Autodesk Fusion 360 part; units mm, degrees
(part 4 of 7)
  arc A299 (52.4822, -27.8177) -> (51.9822, -28.3177) centre (52.4822, -28.3177) ccw
  arc A300 (179.3389, -62.3677) -> (179.8389, -62.8677) centre (179.8389, -62.3677) ccw
  arc A301 (113.1072, -3.7177) -> (113.6072, -3.2177) centre (113.1072, -3.2177) ccw
  arc A302 (-38.5053, -60.3677) -> (-38.0053, -60.8677) centre (-38.0053, -60.3677) ccw
  arc A303 (157.2572, -84.9677) -> (156.7572, -85.4677) centre (157.2572, -85.4677) ccw
  arc A304 (94.5572, 9.7823) -> (94.0572, 10.2823) centre (94.0572, 9.7823) ccw
  arc A305 (46.9322, -28.3177) -> (46.4322, -27.8177) centre (46.4322, -28.3177) ccw
  arc A306 (-52.2928, 10.2823) -> (-52.7928, 9.7823) centre (-52.2928, 9.7823) ccw
  arc A307 (-70.2491, -60.8677) -> (-69.7491, -60.3677) centre (-70.2491, -60.3677) ccw
  arc A308 (-14.1928, -8.7677) -> (-14.6928, -9.2677) centre (-14.1928, -9.2677) ccw
  arc A309 (189.8072, -85.4677) -> (189.3072, -84.9677) centre (189.3072, -85.4677) ccw
  arc A310 (-34.5303, -79.9177) -> (-34.0303, -79.4177) centre (-34.5303, -79.4177) ccw
  arc A311 (75.5072, -9.2677) -> (75.0072, -8.7677) centre (75.0072, -9.2677) ccw
  line L329 (113.6072, 9.7823) -> (113.6072, -3.2177)
  arc A312 (-0.6928, 9.7823) -> (-1.1928, 10.2823) centre (-1.1928, 9.7823) ccw
  arc A313 (208.8572, -85.4677) -> (208.3572, -84.9677) centre (208.3572, -85.4677) ccw
  arc A314 (136.9197, -79.9177) -> (137.4197, -79.4177) centre (136.9197, -79.4177) ccw
  arc A315 (65.9822, -28.3177) -> (65.4822, -27.8177) centre (65.4822, -28.3177) ccw
  arc A316 (75.0072, -3.7177) -> (75.5072, -3.2177) centre (75.0072, -3.2177) ccw
  arc A317 (-15.9491, -100.4677) -> (-15.4491, -100.9677) centre (-15.4491, -100.4677) ccw
  line L330 (114.3947, -60.8677) -> (127.3947, -60.8677)
  arc A318 (195.3572, -84.9677) -> (194.8572, -85.4677) centre (195.3572, -85.4677) ccw
  arc A319 (123.4197, -79.4177) -> (123.9197, -79.9177) centre (123.9197, -79.4177) ccw
  arc A320 (-9.4303, -65.9177) -> (-9.9303, -66.4177) centre (-9.4303, -66.4177) ccw
  line L331 (94.5572, -9.2677) -> (94.5572, -22.2677)
  line L332 (4.3572, -9.2677) -> (4.3572, -22.2677)
  line L333 (-74.5116, -85.4677) -> (-74.5116, -98.4677)
  arc A321 (30.5509, -98.4677) -> (31.0509, -98.9677) centre (31.0509, -98.4677) ccw
  arc A322 (42.4572, -22.2677) -> (42.9572, -22.7677) centre (42.9572, -22.2677) ccw
  arc A323 (-15.4491, -85.9677) -> (-15.9491, -86.4677) centre (-15.4491, -86.4677) ccw
  line L334 (-61.8178, -41.8177) -> (-48.8178, -41.8177)
  line L335 (158.3442, -9.7677) -> (164.3442, -9.7677)
  line L336 (-63.5486, -67.4177) -> (-63.5486, -81.4177)
  line L337 (194.8572, -85.4677) -> (194.8572, -98.4677)
  line L338 (42.1697, -66.4177) -> (42.1697, -79.4177)
  line L339 (99.6072, 9.7823) -> (99.6072, -3.2177)
  arc A324 (100.1072, -8.7677) -> (99.6072, -9.2677) centre (100.1072, -9.2677) ccw
  arc A325 (-57.8428, -9.2677) -> (-58.3428, -8.7677) centre (-58.3428, -9.2677) ccw
  arc A326 (-34.0303, -66.4177) -> (-34.5303, -65.9177) centre (-34.5303, -66.4177) ccw
  arc A327 (-88.5116, -98.4677) -> (-88.0116, -98.9677) centre (-88.0116, -98.4677) ccw
  arc A328 (123.9197, -65.9177) -> (123.4197, -66.4177) centre (123.9197, -66.4177) ccw
  line L340 (75.5072, -9.2677) -> (75.5072, -22.2677)
  line L341 (38.1947, -46.8677) -> (51.1947, -46.8677)
  arc A329 (176.3072, -65.9177) -> (175.8072, -66.4177) centre (176.3072, -66.4177) ccw
  line L342 (-88.0116, -84.9677) -> (-75.0116, -84.9677)
  line L343 (-40.8866, -85.4677) -> (-40.8866, -98.4677)
  line L344 (118.3697, -66.4177) -> (118.3697, -79.4177)
  arc A330 (151.2072, -3.7177) -> (151.7072, -3.2177) centre (151.2072, -3.2177) ccw
  arc A331 (22.6197, -79.9177) -> (23.1197, -79.4177) centre (22.6197, -79.4177) ccw
  arc A332 (-80.4246, -67.4177) -> (-80.9246, -66.9177) centre (-80.9246, -67.4177) ccw
  line L345 (18.3572, -9.2677) -> (18.3572, -22.2677)
  line L346 (-26.8866, -85.4677) -> (-26.8866, -98.4677)
  arc A333 (155.4629, -62.3677) -> (155.9629, -62.8677) centre (155.9629, -62.3677) ccw
  arc A334 (119.1572, -8.7677) -> (118.6572, -9.2677) centre (119.1572, -9.2677) ccw
  arc A335 (-39.2928, -3.7177) -> (-38.7928, -3.2177) centre (-39.2928, -3.2177) ccw
  line L347 (31.0509, -98.9677) -> (44.0509, -98.9677)
  line L348 (-64.9866, -66.4177) -> (-64.9866, -79.4177)
  line L349 (-87.4246, -67.4177) -> (-87.4246, -81.4177)
  arc A336 (17.8572, -22.7677) -> (18.3572, -22.2677) centre (17.8572, -22.2677) ccw
  arc A337 (-83.7491, -60.3677) -> (-83.2491, -60.8677) centre (-83.2491, -60.3677) ccw
  arc A338 (108.3447, -60.8677) -> (108.8447, -60.3677) centre (108.3447, -60.3677) ccw
  line L350 (176.3072, -65.9177) -> (189.3072, -65.9177)
  line L351 (151.7072, 9.7823) -> (151.7072, -3.2177)
  line L352 (-15.9491, -86.4677) -> (-15.9491, -100.4677)
  arc A339 (-52.2928, -8.7677) -> (-52.7928, -9.2677) centre (-52.2928, -9.2677) ccw
  line L353 (-15.4491, -100.9677) -> (-9.4491, -100.9677)
  line L354 (44.5509, -85.4677) -> (44.5509, -98.4677)
  arc A340 (57.2447, -46.8677) -> (56.7447, -47.3677) centre (57.2447, -47.3677) ccw
  arc A341 (85.3197, -79.4177) -> (85.8197, -79.9177) centre (85.8197, -79.4177) ccw
  line L355 (-48.0303, -66.4177) -> (-48.0303, -79.4177)
  line L356 (80.5572, -9.2677) -> (80.5572, -22.2677)
  arc A342 (-15.4803, -79.9177) -> (-14.9803, -79.4177) centre (-15.4803, -79.4177) ccw
  line L357 (56.4572, -9.2677) -> (56.4572, -22.2677)
  line L358 (138.2072, 10.2823) -> (151.2072, 10.2823)
  arc A343 (-74.5116, -85.4677) -> (-75.0116, -84.9677) centre (-75.0116, -85.4677) ccw
  line L359 (156.7572, 9.7823) -> (156.7572, -3.2177)
  line L360 (47.2197, -66.4177) -> (47.2197, -79.4177)
  arc A344 (9.1197, -79.4177) -> (9.6197, -79.9177) centre (9.6197, -79.4177) ccw
  arc A345 (44.0509, -98.9677) -> (44.5509, -98.4677) centre (44.0509, -98.4677) ccw
  line L361 (-50.6991, -85.4677) -> (-50.6991, -98.4677)
  arc A346 (118.6572, -3.2177) -> (119.1572, -3.7177) centre (119.1572, -3.2177) ccw
  line L362 (100.1072, -8.7677) -> (113.1072, -8.7677)
  line L363 (104.3697, -66.4177) -> (104.3697, -79.4177)
  arc A347 (4.8572, -8.7677) -> (4.3572, -9.2677) centre (4.8572, -9.2677) ccw
  line L364 (186.3389, -48.3677) -> (186.3389, -62.3677)
  arc A348 (99.6072, -3.2177) -> (100.1072, -3.7177) centre (100.1072, -3.2177) ccw
  arc A349 (118.3697, -66.4177) -> (117.8697, -65.9177) centre (117.8697, -66.4177) ccw
  line L365 (28.6697, -65.9177) -> (41.6697, -65.9177)
  arc A350 (60.7197, -79.9177) -> (61.2197, -79.4177) centre (60.7197, -79.4177) ccw
  arc A351 (151.7072, 9.7823) -> (151.2072, 10.2823) centre (151.2072, 9.7823) ccw
  arc A352 (51.1947, -60.8677) -> (51.6947, -60.3677) centre (51.1947, -60.3677) ccw
  arc A353 (117.8697, -79.9177) -> (118.3697, -79.4177) centre (117.8697, -79.4177) ccw
  arc A354 (-40.8866, -98.4677) -> (-40.3866, -98.9677) centre (-40.3866, -98.4677) ccw
  arc A355 (-33.2428, 10.2823) -> (-33.7428, 9.7823) centre (-33.2428, 9.7823) ccw
  arc A356 (66.2697, -79.4177) -> (66.7697, -79.9177) centre (66.7697, -79.4177) ccw
  line L366 (157.2572, 10.2823) -> (170.2572, 10.2823)
  arc A357 (176.3072, -84.9677) -> (175.8072, -85.4677) centre (176.3072, -85.4677) ccw
  arc A358 (-64.1991, -84.9677) -> (-64.6991, -85.4677) centre (-64.1991, -85.4677) ccw
  arc A359 (-64.9866, -66.4177) -> (-65.4866, -65.9177) centre (-65.4866, -66.4177) ccw
  line L367 (-80.4246, -67.4177) -> (-80.4246, -81.4177)
  arc A360 (3.5697, -79.9177) -> (4.0697, -79.4177) centre (3.5697, -79.4177) ccw
  arc A361 (-58.3428, -3.7177) -> (-57.8428, -3.2177) centre (-58.3428, -3.2177) ccw
  arc A362 (-28.4803, -65.9177) -> (-28.9803, -66.4177) centre (-28.4803, -66.4177) ccw
  line L368 (100.1072, -3.7177) -> (113.1072, -3.7177)
  arc A363 (-5.9553, -60.8677) -> (-5.4553, -60.3677) centre (-5.9553, -60.3677) ccw
  arc A364 (-88.0116, -84.9677) -> (-88.5116, -85.4677) centre (-88.0116, -85.4677) ccw
  line L369 (37.4072, -9.2677) -> (37.4072, -22.2677)
  arc A365 (51.6947, -47.3677) -> (51.1947, -46.8677) centre (51.1947, -47.3677) ccw
  arc A366 (19.1447, -46.8677) -> (18.6447, -47.3677) centre (19.1447, -47.3677) ccw
  arc A367 (51.9822, -41.3177) -> (52.4822, -41.8177) centre (52.4822, -41.3177) ccw
  line L370 (99.3197, -66.4177) -> (99.3197, -79.4177)
  line L371 (-19.7428, -9.2677) -> (-19.7428, -22.2677)
  line L372 (47.7197, -65.9177) -> (60.7197, -65.9177)
  line L373 (52.4822, -41.8177) -> (65.4822, -41.8177)
  line L374 (52.4822, -27.8177) -> (65.4822, -27.8177)
  arc A368 (170.2572, -3.7177) -> (170.7572, -3.2177) centre (170.2572, -3.2177) ccw
  line L375 (189.8072, 9.7823) -> (189.8072, -3.2177)
  arc A369 (180.2822, -9.2677) -> (179.7822, -8.7677) centre (179.7822, -9.2677) ccw
  line L376 (208.8572, 9.7823) -> (208.8572, -3.2177)
  arc A370 (208.8572, 9.7823) -> (208.3572, 10.2823) centre (208.3572, 9.7823) ccw
  arc A371 (195.3572, 10.2823) -> (194.8572, 9.7823) centre (195.3572, 9.7823) ccw
  arc A372 (182.2202, -9.7677) -> (181.7202, -10.2677) centre (182.2202, -10.2677) ccw
  arc A373 (208.3572, -3.7177) -> (208.8572, -3.2177) centre (208.3572, -3.2177) ccw
  line L377 (195.3572, 10.2823) -> (208.3572, 10.2823)
  line L378 (195.3572, -3.7177) -> (208.3572, -3.7177)
  line L379 (176.3072, -3.7177) -> (189.3072, -3.7177)
  line L380 (176.3072, 10.2823) -> (189.3072, 10.2823)
  arc A374 (175.8072, -3.2177) -> (176.3072, -3.7177) centre (176.3072, -3.2177) ccw
  arc A375 (195.3572, -8.7677) -> (194.8572, -9.2677) centre (195.3572, -9.2677) ccw
  arc A376 (176.3072, 10.2823) -> (175.8072, 9.7823) centre (176.3072, 9.7823) ccw
  line L381 (195.3572, -8.7677) -> (208.3572, -8.7677)
  arc A377 (170.7572, 9.7823) -> (170.2572, 10.2823) centre (170.2572, 9.7823) ccw
  arc A378 (177.9009, -47.3677) -> (177.4009, -46.8677) centre (177.4009, -47.3677) ccw
  arc A379 (208.8572, -28.3177) -> (208.3572, -27.8177) centre (208.3572, -28.3177) ccw
  arc A380 (171.5447, -27.8177) -> (171.0447, -28.3177) centre (171.5447, -28.3177) ccw
  line L382 (146.9447, -47.3677) -> (146.9447, -60.3677)
  arc A381 (188.2202, -24.7677) -> (188.7202, -24.2677) centre (188.2202, -24.2677) ccw
  line L383 (171.0447, -28.3177) -> (171.0447, -41.3177)
  line L384 (-5.4553, -47.3677) -> (-5.4553, -60.3677)
  arc A382 (195.3572, -27.8177) -> (194.8572, -28.3177) centre (195.3572, -28.3177) ccw
  arc A383 (162.4629, -48.3677) -> (161.9629, -47.8677) centre (161.9629, -48.3677) ccw
  line L385 (208.8572, -9.2677) -> (208.8572, -22.2677)
  line L386 (132.9447, -47.3677) -> (132.9447, -60.3677)
  arc A384 (195.3572, -46.8677) -> (194.8572, -47.3677) centre (195.3572, -47.3677) ccw
  line L387 (180.2822, -9.2677) -> (180.2822, -22.2677)
  arc A385 (186.3389, -48.3677) -> (185.8389, -47.8677) centre (185.8389, -48.3677) ccw
  line L388 (181.7202, -10.2677) -> (181.7202, -24.2677)
  line L389 (-24.5053, -47.3677) -> (-24.5053, -60.3677)
  line L390 (-113.7226, -118.8427) -> (-113.7226, 57.4273)
  line L391 (42.9572, 10.2823) -> (55.9572, 10.2823)
  line L392 (188.7202, -10.2677) -> (188.7202, -24.2677)
  arc A386 (37.4072, -9.2677) -> (36.9072, -8.7677) centre (36.9072, -9.2677) ccw
  line L393 (-43.5553, -47.3677) -> (-43.5553, -60.3677)
  line L394 (194.8572, -9.2677) -> (194.8572, -22.2677)
  line L395 (75.7947, -47.3677) -> (75.7947, -60.3677)
  line L396 (-57.5553, -47.3677) -> (-57.5553, -60.3677)
  line L397 (194.8572, -47.3677) -> (194.8572, -60.3677)
  line L398 (42.9572, -3.7177) -> (55.9572, -3.7177)
  line L399 (177.9009, -47.3677) -> (177.9009, -60.3677)
  arc A387 (55.9572, -3.7177) -> (56.4572, -3.2177) centre (55.9572, -3.2177) ccw
  arc A388 (56.4572, 9.7823) -> (55.9572, 10.2823) centre (55.9572, 9.7823) ccw
  arc A389 (17.8572, -3.7177) -> (18.3572, -3.2177) centre (17.8572, -3.2177) ccw
  line L400 (194.8572, 9.7823) -> (194.8572, -3.2177)
  arc A390 (194.8572, -3.2177) -> (195.3572, -3.7177) centre (195.3572, -3.2177) ccw
  line L401 (175.8072, 9.7823) -> (175.8072, -3.2177)
  arc A391 (188.7202, -10.2677) -> (188.2202, -9.7677) centre (188.2202, -10.2677) ccw
  arc A392 (208.8572, -47.3677) -> (208.3572, -46.8677) centre (208.3572, -47.3677) ccw
  line L402 (171.5447, -27.8177) -> (184.5447, -27.8177)
  arc A393 (179.7822, -22.7677) -> (180.2822, -22.2677) centre (179.7822, -22.2677) ccw
  line L403 (163.9009, -47.3677) -> (163.9009, -60.3677)
  line L404 (195.3572, -46.8677) -> (208.3572, -46.8677)
  line L405 (94.8447, -47.3677) -> (94.8447, -60.3677)
  line L406 (182.2202, -24.7677) -> (188.2202, -24.7677)
  line L407 (179.8389, -47.8677) -> (185.8389, -47.8677)
  line L408 (208.8572, -28.3177) -> (208.8572, -41.3177)
  arc A394 (184.5447, -41.8177) -> (185.0447, -41.3177) centre (184.5447, -41.3177) ccw
  arc A395 (185.0447, -28.3177) -> (184.5447, -27.8177) centre (184.5447, -28.3177) ccw
  arc A396 (189.3072, -3.7177) -> (189.8072, -3.2177) centre (189.3072, -3.2177) ccw
  arc A397 (189.8072, 9.7823) -> (189.3072, 10.2823) centre (189.3072, 9.7823) ccw
  line L409 (182.2202, -9.7677) -> (188.2202, -9.7677)
  line L410 (47.7197, -79.9177) -> (60.7197, -79.9177)
  line L411 (57.2447, -46.8677) -> (70.2447, -46.8677)
  line L412 (-113.7226, 57.4273) -> (228.9474, 57.4273)
  line L413 (18.6447, -47.3677) -> (18.6447, -60.3677)
  line L414 (89.7947, -47.3677) -> (89.7947, -60.3677)
  arc A398 (36.9072, -3.7177) -> (37.4072, -3.2177) centre (36.9072, -3.2177) ccw
  arc A399 (42.9572, -8.7677) -> (42.4572, -9.2677) centre (42.9572, -9.2677) ccw
  line L415 (56.7447, -47.3677) -> (56.7447, -60.3677)
  line L416 (51.6947, -47.3677) -> (51.6947, -60.3677)
  line L417 (-0.4053, -47.3677) -> (-0.4053, -60.3677)
  line L418 (208.8572, -47.3677) -> (208.8572, -60.3677)
  arc A400 (37.4072, 9.7823) -> (36.9072, 10.2823) centre (36.9072, 9.7823) ccw
  line L419 (13.5947, -47.3677) -> (13.5947, -60.3677)
  line L420 (-83.7491, -47.3677) -> (-83.7491, -60.3677)
  line L421 (-38.5053, -47.3677) -> (-38.5053, -60.3677)
  line L422 (127.8947, -47.3677) -> (127.8947, -60.3677)
  line L423 (37.6947, -47.3677) -> (37.6947, -60.3677)
  arc A401 (23.9072, -8.7677) -> (23.4072, -9.2677) centre (23.9072, -9.2677) ccw
  arc A402 (179.8389, -47.8677) -> (179.3389, -48.3677) centre (179.8389, -48.3677) ccw
  line L424 (70.7447, -47.3677) -> (70.7447, -60.3677)
  line L425 (-19.4553, -47.3677) -> (-19.4553, -60.3677)
  arc A403 (56.4572, -9.2677) -> (55.9572, -8.7677) centre (55.9572, -9.2677) ccw
  line L426 (113.8947, -47.3677) -> (113.8947, -60.3677)
  arc A404 (23.9072, 10.2823) -> (23.4072, 9.7823) centre (23.9072, 9.7823) ccw
  line L427 (108.8447, -47.3677) -> (108.8447, -60.3677)
  line L428 (-69.7491, -47.3677) -> (-69.7491, -60.3677)
  line L429 (32.6447, -47.3677) -> (32.6447, -60.3677)
  line L430 (-18.9553, -60.8677) -> (-5.9553, -60.8677)
  line L431 (-23.7178, -27.8177) -> (-10.7178, -27.8177)
  line L432 (228.9474, 57.4273) -> (228.9474, -118.8427)
  arc A405 (18.3572, -9.2677) -> (17.8572, -8.7677) centre (17.8572, -9.2677) ccw
  line L433 (-28.4803, -65.9177) -> (-15.4803, -65.9177)
  line L434 (-33.2428, 10.2823) -> (-20.2428, 10.2823)
  arc A406 (42.4572, -3.2177) -> (42.9572, -3.7177) centre (42.9572, -3.2177) ccw
  line L435 (23.9072, -8.7677) -> (36.9072, -8.7677)
  line L436 (-33.2428, -8.7677) -> (-20.2428, -8.7677)
  line L437 (42.4572, 9.7823) -> (42.4572, -3.2177)
  line L438 (-23.7178, -41.8177) -> (-10.7178, -41.8177)
  line L439 (18.3572, 9.7823) -> (18.3572, -3.2177)
  line L440 (119.1572, -8.7677) -> (132.1572, -8.7677)
  arc A407 (155.9629, -47.8677) -> (155.4629, -48.3677) centre (155.9629, -48.3677) ccw
  line L441 (-28.4803, -79.9177) -> (-15.4803, -79.9177)
  line L442 (123.9197, -79.9177) -> (136.9197, -79.9177)
  line L443 (-57.0553, -60.8677) -> (-44.0553, -60.8677)
  line L444 (128.6822, -27.8177) -> (141.6822, -27.8177)
  line L445 (-64.1991, -98.9677) -> (-51.1991, -98.9677)
  line L446 (-64.1991, -84.9677) -> (-51.1991, -84.9677)
  line L447 (128.6822, -41.8177) -> (141.6822, -41.8177)
  line L448 (42.9572, -8.7677) -> (55.9572, -8.7677)
  line L449 (9.6197, -79.9177) -> (22.6197, -79.9177)
  line L450 (19.1447, -60.8677) -> (32.1447, -60.8677)
  line L451 (-33.2428, -22.7677) -> (-20.2428, -22.7677)
  line L452 (133.4447, -60.8677) -> (146.4447, -60.8677)
  arc A408 (157.2572, 10.2823) -> (156.7572, 9.7823) centre (157.2572, 9.7823) ccw
  line L453 (123.9197, -65.9177) -> (136.9197, -65.9177)
  line L454 (9.6197, -65.9177) -> (22.6197, -65.9177)
  line L455 (119.1572, -22.7677) -> (132.1572, -22.7677)
  line L456 (119.1572, -3.7177) -> (132.1572, -3.7177)
  line L457 (28.6697, -79.9177) -> (41.6697, -79.9177)
  line L458 (119.1572, 10.2823) -> (132.1572, 10.2823)
  line L459 (85.8197, -65.9177) -> (98.8197, -65.9177)
  line L460 (37.4072, 9.7823) -> (37.4072, -3.2177)
  line L461 (138.2072, -8.7677) -> (151.2072, -8.7677)
  line L462 (4.8572, -8.7677) -> (17.8572, -8.7677)
  line L463 (-9.4303, -79.9177) -> (3.5697, -79.9177)
  line L464 (-9.9303, -66.4177) -> (-9.9303, -79.4177)
  arc A409 (-44.0553, -60.8677) -> (-43.5553, -60.3677) centre (-44.0553, -60.3677) ccw
  line L465 (-78.9866, -66.4177) -> (-78.9866, -79.4177)
  line L466 (-15.4491, -85.9677) -> (-9.4491, -85.9677)
  line L467 (-86.9246, -66.9177) -> (-80.9246, -66.9177)
  arc A410 (132.6572, -9.2677) -> (132.1572, -8.7677) centre (132.1572, -9.2677) ccw
  arc A411 (85.8197, -65.9177) -> (85.3197, -66.4177) centre (85.8197, -66.4177) ccw
  arc A412 (-64.6991, -98.4677) -> (-64.1991, -98.9677) centre (-64.1991, -98.4677) ccw
  arc A413 (28.1697, -79.4177) -> (28.6697, -79.9177) centre (28.6697, -79.4177) ccw
  arc A414 (-56.5486, -67.4177) -> (-57.0486, -66.9177) centre (-57.0486, -67.4177) ccw
  arc A415 (56.7447, -60.3677) -> (57.2447, -60.8677) centre (57.2447, -60.3677) ccw
  line L468 (-71.3428, 10.2823) -> (-58.3428, 10.2823)
  line L469 (-9.4303, -65.9177) -> (3.5697, -65.9177)
  arc A416 (156.7572, -3.2177) -> (157.2572, -3.7177) centre (157.2572, -3.2177) ccw
  line L470 (4.8572, 10.2823) -> (17.8572, 10.2823)
  line L471 (31.0509, -84.9677) -> (44.0509, -84.9677)
  line L472 (-88.0116, -98.9677) -> (-75.0116, -98.9677)
  arc A417 (32.1447, -60.8677) -> (32.6447, -60.3677) centre (32.1447, -60.3677) ccw
  arc A418 (44.5509, -85.4677) -> (44.0509, -84.9677) centre (44.0509, -85.4677) ccw
  line L473 (56.4572, 9.7823) -> (56.4572, -3.2177)
  arc A419 (189.3072, -79.9177) -> (189.8072, -79.4177) centre (189.3072, -79.4177) ccw
  arc A420 (-28.9803, -79.4177) -> (-28.4803, -79.9177) centre (-28.4803, -79.4177) ccw
  line L474 (28.1697, -66.4177) -> (28.1697, -79.4177)
  arc A421 (175.8072, -79.4177) -> (176.3072, -79.9177) centre (176.3072, -79.4177) ccw
  arc A422 (66.7697, -65.9177) -> (66.2697, -66.4177) centre (66.7697, -66.4177) ccw
  arc A423 (99.3197, -66.4177) -> (98.8197, -65.9177) centre (98.8197, -66.4177) ccw
  arc A424 (47.2197, -79.4177) -> (47.7197, -79.9177) centre (47.7197, -79.4177) ccw
  line L475 (23.4072, -9.2677) -> (23.4072, -22.2677)
  line L476 (-47.5303, -65.9177) -> (-34.5303, -65.9177)
  arc A425 (37.6947, -60.3677) -> (38.1947, -60.8677) centre (38.1947, -60.3677) ccw
  arc A426 (23.1197, -66.4177) -> (22.6197, -65.9177) centre (22.6197, -66.4177) ccw
  arc A427 (137.7072, -3.2177) -> (138.2072, -3.7177) centre (138.2072, -3.2177) ccw
  arc A428 (208.3572, -79.9177) -> (208.8572, -79.4177) centre (208.3572, -79.4177) ccw
  arc A429 (-63.0486, -66.9177) -> (-63.5486, -67.4177) centre (-63.0486, -67.4177) ccw
  line L477 (99.6072, -9.2677) -> (99.6072, -22.2677)
  line L478 (30.5509, -85.4677) -> (30.5509, -98.4677)
  arc A430 (194.8572, -79.4177) -> (195.3572, -79.9177) centre (195.3572, -79.4177) ccw
  arc A431 (31.0509, -84.9677) -> (30.5509, -85.4677) centre (31.0509, -85.4677) ccw
  arc A432 (-86.9246, -66.9177) -> (-87.4246, -67.4177) centre (-86.9246, -67.4177) ccw
  arc A433 (-14.9803, -66.4177) -> (-15.4803, -65.9177) centre (-15.4803, -66.4177) ccw
  line L479 (-28.9803, -66.4177) -> (-28.9803, -79.4177)
  line L480 (138.2072, -3.7177) -> (151.2072, -3.7177)
  line L481 (0.0947, -60.8677) -> (13.0947, -60.8677)
  arc A434 (-75.0116, -98.9677) -> (-74.5116, -98.4677) centre (-75.0116, -98.4677) ccw
  arc A435 (42.1697, -66.4177) -> (41.6697, -65.9177) centre (41.6697, -66.4177) ccw
  arc A436 (158.3442, -9.7677) -> (157.8442, -10.2677) centre (158.3442, -10.2677) ccw
  arc A437 (132.9447, -60.3677) -> (133.4447, -60.8677) centre (133.4447, -60.3677) ccw
  line L482 (-63.0486, -81.9177) -> (-57.0486, -81.9177)
  line L483 (-14.6928, -9.2677) -> (-14.6928, -22.2677)
  line L484 (-88.5116, -85.4677) -> (-88.5116, -98.4677)
  line L485 (164.4009, -46.8677) -> (177.4009, -46.8677)
  line L486 (-86.9246, -81.9177) -> (-80.9246, -81.9177)
  line L487 (23.1197, -66.4177) -> (23.1197, -79.4177)
  arc A438 (-0.4053, -60.3677) -> (0.0947, -60.8677) centre (0.0947, -60.3677) ccw
  arc A439 (98.8197, -79.9177) -> (99.3197, -79.4177) centre (98.8197, -79.4177) ccw
  line L488 (61.5072, -9.2677) -> (61.5072, -22.2677)
  line L489 (-64.6991, -85.4677) -> (-64.6991, -98.4677)
  arc A440 (-65.4866, -79.9177) -> (-64.9866, -79.4177) centre (-65.4866, -79.4177) ccw
  arc A441 (132.6572, 9.7823) -> (132.1572, 10.2823) centre (132.1572, 9.7823) ccw
  arc A442 (-27.3866, -98.9677) -> (-26.8866, -98.4677) centre (-27.3866, -98.4677) ccw
  arc A443 (47.7197, -65.9177) -> (47.2197, -66.4177) centre (47.7197, -66.4177) ccw
  arc A444 (138.2072, -8.7677) -> (137.7072, -9.2677) centre (138.2072, -9.2677) ccw
  arc A445 (18.3572, 9.7823) -> (17.8572, 10.2823) centre (17.8572, 9.7823) ccw
  arc A446 (28.6697, -65.9177) -> (28.1697, -66.4177) centre (28.6697, -66.4177) ccw
  line L490 (-71.3428, -8.7677) -> (-58.3428, -8.7677)
  line L491 (-71.3428, -3.7177) -> (-58.3428, -3.7177)
  arc A447 (42.9572, 10.2823) -> (42.4572, 9.7823) centre (42.9572, 9.7823) ccw
  line L492 (164.4009, -60.8677) -> (177.4009, -60.8677)
  line L493 (81.0572, 10.2823) -> (94.0572, 10.2823)
  line L494 (157.2572, -3.7177) -> (170.2572, -3.7177)
  line L495 (81.0572, -8.7677) -> (94.0572, -8.7677)
  line L496 (38.1947, -60.8677) -> (51.1947, -60.8677)
  arc A448 (132.1572, -3.7177) -> (132.6572, -3.2177) centre (132.1572, -3.2177) ccw
  arc A449 (-87.4246, -81.4177) -> (-86.9246, -81.9177) centre (-86.9246, -81.4177) ccw
  arc A450 (164.8442, -10.2677) -> (164.3442, -9.7677) centre (164.3442, -10.2677) ccw
  arc A451 (-8.9491, -86.4677) -> (-9.4491, -85.9677) centre (-9.4491, -86.4677) ccw
  arc A452 (13.0947, -60.8677) -> (13.5947, -60.3677) centre (13.0947, -60.3677) ccw
  line L497 (95.3447, -60.8677) -> (108.3447, -60.8677)
  line L498 (-38.0053, -60.8677) -> (-25.0053, -60.8677)
  arc A453 (-80.9246, -81.9177) -> (-80.4246, -81.4177) centre (-80.9246, -81.4177) ccw
  line L499 (90.5822, -27.8177) -> (103.5822, -27.8177)
  arc A454 (-57.0486, -81.9177) -> (-56.5486, -81.4177) centre (-57.0486, -81.4177) ccw
  line L500 (166.7822, -8.7677) -> (179.7822, -8.7677)
  line L501 (-33.2428, -3.7177) -> (-20.2428, -3.7177)
  line L502 (132.6572, 9.7823) -> (132.6572, -3.2177)
  line L503 (23.4072, 9.7823) -> (23.4072, -3.2177)
  line L504 (-61.8178, -27.8177) -> (-48.8178, -27.8177)
  line L505 (81.0572, -3.7177) -> (94.0572, -3.7177)
  line L506 (23.9072, -3.7177) -> (36.9072, -3.7177)
  arc A455 (41.6697, -79.9177) -> (42.1697, -79.4177) centre (41.6697, -79.4177) ccw
  line L507 (90.5822, -41.8177) -> (103.5822, -41.8177)
  arc A456 (-63.5486, -81.4177) -> (-63.0486, -81.9177) centre (-63.0486, -81.4177) ccw
  line L508 (-40.3866, -98.9677) -> (-27.3866, -98.9677)
  arc A457 (-25.0053, -60.8677) -> (-24.5053, -60.3677) centre (-25.0053, -60.3677) ccw
  line L509 (137.7072, 9.7823) -> (137.7072, -3.2177)
  line L510 (4.8572, -3.7177) -> (17.8572, -3.7177)
  line L511 (14.3822, -41.8177) -> (27.3822, -41.8177)
  line L512 (4.8572, -22.7677) -> (17.8572, -22.7677)
  arc A458 (23.4072, -3.2177) -> (23.9072, -3.7177) centre (23.9072, -3.2177) ccw
  line L513 (-47.5303, -79.9177) -> (-34.5303, -79.9177)
  line L514 (85.8197, -79.9177) -> (98.8197, -79.9177)
  line L515 (81.0572, -22.7677) -> (94.0572, -22.7677)
  line L516 (-56.5486, -67.4177) -> (-56.5486, -81.4177)
  arc A459 (-9.9303, -79.4177) -> (-9.4303, -79.9177) centre (-9.4303, -79.4177) ccw
  line L517 (23.9072, 10.2823) -> (36.9072, 10.2823)
  line L518 (-34.0303, -66.4177) -> (-34.0303, -79.4177)
  line L519 (14.3822, -27.8177) -> (27.3822, -27.8177)
  arc A460 (194.8572, -41.3177) -> (195.3572, -41.8177) centre (195.3572, -41.3177) ccw
  arc A461 (194.8572, -22.2677) -> (195.3572, -22.7677) centre (195.3572, -22.2677) ccw
  line L520 (194.8572, -28.3177) -> (194.8572, -41.3177)
  line L521 (195.3572, -22.7677) -> (208.3572, -22.7677)
  arc A462 (208.3572, -41.8177) -> (208.8572, -41.3177) centre (208.3572, -41.3177) ccw
  line L522 (185.0447, -28.3177) -> (185.0447, -41.3177)
  line L523 (195.3572, -41.8177) -> (208.3572, -41.8177)
  arc A463 (181.7202, -24.2677) -> (182.2202, -24.7677) centre (182.2202, -24.2677) ccw
  arc A464 (208.3572, -22.7677) -> (208.8572, -22.2677) centre (208.3572, -22.2677) ccw
  line L524 (171.5447, -41.8177) -> (184.5447, -41.8177)
  arc A465 (171.0447, -41.3177) -> (171.5447, -41.8177) centre (171.5447, -41.3177) ccw
  line L525 (195.3572, -27.8177) -> (208.3572, -27.8177)
  line L526 (57.2447, -60.8677) -> (70.2447, -60.8677)
  line L527 (228.9474, -118.8427) -> (-113.7226, -118.8427)
  line L528 (123.1322, -28.3177) -> (123.1322, -41.3177)
  arc A466 (114.3947, -46.8677) -> (113.8947, -47.3677) centre (114.3947, -47.3677) ccw
  line L529 (156.7572, -85.4677) -> (156.7572, -98.4677)
  line L530 (151.7072, -85.4677) -> (151.7072, -98.4677)
  arc A467 (-71.8428, -22.2677) -> (-71.3428, -22.7677) centre (-71.3428, -22.2677) ccw
  line L531 (-57.0553, -46.8677) -> (-44.0553, -46.8677)
  arc A468 (-69.7491, -47.3677) -> (-70.2491, -46.8677) centre (-70.2491, -47.3677) ccw
  arc A469 (-90.8928, -22.2677) -> (-90.3928, -22.7677) centre (-90.3928, -22.2677) ccw
  arc A470 (170.2572, -98.9677) -> (170.7572, -98.4677) centre (170.2572, -98.4677) ccw
  arc A471 (-86.1303, -41.3177) -> (-85.6303, -41.8177) centre (-85.6303, -41.3177) ccw
  arc A472 (149.6134, -79.4177) -> (150.1134, -79.9177) centre (150.1134, -79.4177) ccw
  arc A473 (-85.6303, -27.8177) -> (-86.1303, -28.3177) centre (-85.6303, -28.3177) ccw
  line L532 (8.8322, -28.3177) -> (8.8322, -41.3177)
  arc A474 (-77.3928, -22.7677) -> (-76.8928, -22.2677) centre (-77.3928, -22.2677) ccw
  line L533 (95.3447, -46.8677) -> (108.3447, -46.8677)
  line L534 (-29.2678, -28.3177) -> (-29.2678, -41.3177)
  arc A475 (-38.0053, -46.8677) -> (-38.5053, -47.3677) centre (-38.0053, -47.3677) ccw
  line L535 (-85.6303, -27.8177) -> (-72.6303, -27.8177)
  arc A476 (163.1134, -79.9177) -> (163.6134, -79.4177) centre (163.1134, -79.4177) ccw
  arc A477 (-33.7428, -22.2677) -> (-33.2428, -22.7677) centre (-33.2428, -22.2677) ccw
  line L536 (114.3947, -46.8677) -> (127.3947, -46.8677)
  arc A478 (14.3822, -27.8177) -> (13.8822, -28.3177) centre (14.3822, -28.3177) ccw
  arc A479 (-58.3428, -22.7677) -> (-57.8428, -22.2677) centre (-58.3428, -22.2677) ccw
  arc A480 (161.9629, -62.8677) -> (162.4629, -62.3677) centre (161.9629, -62.3677) ccw
  line L537 (-85.6303, -41.8177) -> (-72.6303, -41.8177)
  arc A481 (-42.7678, -27.8177) -> (-43.2678, -28.3177) centre (-42.7678, -28.3177) ccw
  arc A482 (163.9009, -60.3677) -> (164.4009, -60.8677) centre (164.4009, -60.3677) ccw
  line L538 (-18.9553, -46.8677) -> (-5.9553, -46.8677)
  arc A483 (-29.2678, -28.3177) -> (-29.7678, -27.8177) centre (-29.7678, -28.3177) ccw
  arc A484 (-4.6678, -27.8177) -> (-5.1678, -28.3177) centre (-4.6678, -28.3177) ccw
  line L539 (137.4197, -66.4177) -> (137.4197, -79.4177)
  line L540 (163.6134, -66.4177) -> (163.6134, -79.4177)
  arc A485 (-83.2491, -46.8677) -> (-83.7491, -47.3677) centre (-83.2491, -47.3677) ccw
  arc A486 (146.4447, -60.8677) -> (146.9447, -60.3677) centre (146.4447, -60.3677) ccw
  line L541 (170.7572, -85.4677) -> (170.7572, -98.4677)
  line L542 (157.2572, -84.9677) -> (170.2572, -84.9677)
  arc A487 (-39.2928, -22.7677) -> (-38.7928, -22.2677) centre (-39.2928, -22.2677) ccw
  arc A488 (-24.2178, -41.3177) -> (-23.7178, -41.8177) centre (-23.7178, -41.3177) ccw
  arc A489 (-29.7678, -41.8177) -> (-29.2678, -41.3177) centre (-29.7678, -41.3177) ccw
  arc A490 (-48.8178, -41.8177) -> (-48.3178, -41.3177) centre (-48.8178, -41.3177) ccw
  arc A491 (151.2072, -98.9677) -> (151.7072, -98.4677) centre (151.2072, -98.4677) ccw
  arc A492 (-43.5553, -47.3677) -> (-44.0553, -46.8677) centre (-44.0553, -47.3677) ccw
  arc A493 (208.8572, -9.2677) -> (208.3572, -8.7677) centre (208.3572, -9.2677) ccw
  line L543 (170.7572, 9.7823) -> (170.7572, -3.2177)
  arc A494 (-72.1303, -28.3177) -> (-72.6303, -27.8177) centre (-72.6303, -28.3177) ccw
  arc A495 (0.0947, -46.8677) -> (-0.4053, -47.3677) centre (0.0947, -47.3677) ccw
  arc A496 (122.6322, -41.8177) -> (123.1322, -41.3177) centre (122.6322, -41.3177) ccw
  line L544 (13.8822, -28.3177) -> (13.8822, -41.3177)
  line L545 (155.9629, -62.8677) -> (161.9629, -62.8677)
  line L546 (147.7322, -27.8177) -> (160.7322, -27.8177)
  arc A497 (-62.3178, -41.3177) -> (-61.8178, -41.8177) centre (-61.8178, -41.3177) ccw
  line L547 (147.2322, -28.3177) -> (147.2322, -41.3177)
  line L548 (71.5322, -27.8177) -> (84.5322, -27.8177)
  line L549 (133.4447, -46.8677) -> (146.4447, -46.8677)
  line L550 (0.0947, -46.8677) -> (13.0947, -46.8677)
  line L551 (158.3442, -24.7677) -> (164.3442, -24.7677)
  arc A498 (-90.3928, 10.2823) -> (-90.8928, 9.7823) centre (-90.3928, 9.7823) ccw
  line L552 (-90.8928, 9.7823) -> (-90.8928, -3.2177)
  line L553 (-10.2178, -28.3177) -> (-10.2178, -41.3177)
  line L554 (100.1072, -22.7677) -> (113.1072, -22.7677)
  arc A499 (89.7947, -47.3677) -> (89.2947, -46.8677) centre (89.2947, -47.3677) ccw
  line L555 (-90.3928, 10.2823) -> (-77.3928, 10.2823)
  line L556 (-62.3178, -28.3177) -> (-62.3178, -41.3177)
  arc A500 (118.6572, -22.2677) -> (119.1572, -22.7677) centre (119.1572, -22.2677) ccw
  arc A501 (109.1322, -41.3177) -> (109.6322, -41.8177) centre (109.6322, -41.3177) ccw
  arc A502 (123.1322, -28.3177) -> (122.6322, -27.8177) centre (122.6322, -28.3177) ccw
  line L557 (137.7072, -85.4677) -> (137.7072, -98.4677)
  arc A503 (-52.7928, -22.2677) -> (-52.2928, -22.7677) centre (-52.2928, -22.2677) ccw
  line L558 (61.2197, -66.4177) -> (61.2197, -79.4177)
  line L559 (-71.8428, 9.7823) -> (-71.8428, -3.2177)
  line L560 (147.7322, -41.8177) -> (160.7322, -41.8177)
  arc A504 (113.1072, -22.7677) -> (113.6072, -22.2677) centre (113.1072, -22.2677) ccw
  arc A505 (142.1822, -28.3177) -> (141.6822, -27.8177) centre (141.6822, -28.3177) ccw
  line L561 (-43.2678, -28.3177) -> (-43.2678, -41.3177)
  arc A506 (-76.8928, -9.2677) -> (-77.3928, -8.7677) centre (-77.3928, -9.2677) ccw
  arc A507 (-48.3178, -28.3177) -> (-48.8178, -27.8177) centre (-48.8178, -28.3177) ccw
  line L562 (-90.3928, -8.7677) -> (-77.3928, -8.7677)
  arc A508 (104.0822, -28.3177) -> (103.5822, -27.8177) centre (103.5822, -28.3177) ccw
  line L563 (-14.1928, -22.7677) -> (-1.1928, -22.7677)
  arc A509 (156.7572, -98.4677) -> (157.2572, -98.9677) centre (157.2572, -98.4677) ccw
  arc A510 (-43.2678, -41.3177) -> (-42.7678, -41.8177) centre (-42.7678, -41.3177) ccw
  arc A511 (-18.9553, -46.8677) -> (-19.4553, -47.3677) centre (-18.9553, -47.3677) ccw
  arc A512 (-23.7178, -27.8177) -> (-24.2178, -28.3177) centre (-23.7178, -28.3177) ccw
  line L564 (-42.7678, -27.8177) -> (-29.7678, -27.8177)
  line L565 (-90.3928, -3.7177) -> (-77.3928, -3.7177)
  arc A513 (-77.3928, -3.7177) -> (-76.8928, -3.2177) centre (-77.3928, -3.2177) ccw
  arc A514 (13.5947, -47.3677) -> (13.0947, -46.8677) centre (13.0947, -47.3677) ccw
  arc A515 (-90.3928, -8.7677) -> (-90.8928, -9.2677) centre (-90.3928, -9.2677) ccw
  arc A516 (141.6822, -41.8177) -> (142.1822, -41.3177) centre (141.6822, -41.3177) ccw
  arc A517 (-61.8178, -27.8177) -> (-62.3178, -28.3177) centre (-61.8178, -28.3177) ccw
  arc A518 (164.3442, -24.7677) -> (164.8442, -24.2677) centre (164.3442, -24.2677) ccw
  arc A519 (-14.6928, -22.2677) -> (-14.1928, -22.7677) centre (-14.1928, -22.2677) ccw
  arc A520 (94.0572, -22.7677) -> (94.5572, -22.2677) centre (94.0572, -22.2677) ccw
  arc A521 (-90.8928, -3.2177) -> (-90.3928, -3.7177) centre (-90.3928, -3.2177) ccw
  arc A522 (-71.3428, -8.7677) -> (-71.8428, -9.2677) centre (-71.3428, -9.2677) ccw
  line L566 (161.2322, -28.3177) -> (161.2322, -41.3177)
  arc A523 (-72.6303, -41.8177) -> (-72.1303, -41.3177) centre (-72.6303, -41.3177) ccw
  arc A524 (128.6822, -27.8177) -> (128.1822, -28.3177) centre (128.6822, -28.3177) ccw
  arc A525 (170.7572, -85.4677) -> (170.2572, -84.9677) centre (170.2572, -85.4677) ccw
  arc A526 (13.8822, -41.3177) -> (14.3822, -41.8177) centre (14.3822, -41.3177) ccw
  line L567 (109.6322, -27.8177) -> (122.6322, -27.8177)
  line L568 (104.0822, -28.3177) -> (104.0822, -41.3177)
  arc A527 (99.6072, -22.2677) -> (100.1072, -22.7677) centre (100.1072, -22.2677) ccw
  arc A528 (164.4009, -46.8677) -> (163.9009, -47.3677) centre (164.4009, -47.3677) ccw
  line L569 (-90.3928, -22.7677) -> (-77.3928, -22.7677)
  line L570 (-76.8928, 9.7823) -> (-76.8928, -3.2177)
  arc A529 (8.3322, -41.8177) -> (8.8322, -41.3177) centre (8.3322, -41.3177) ccw
  arc A530 (-71.3428, 10.2823) -> (-71.8428, 9.7823) centre (-71.3428, 9.7823) ccw
  line L571 (100.1072, 10.2823) -> (113.1072, 10.2823)
  arc A531 (81.0572, -8.7677) -> (80.5572, -9.2677) centre (81.0572, -9.2677) ccw
  arc A532 (189.3072, -98.9677) -> (189.8072, -98.4677) centre (189.3072, -98.4677) ccw
  line L572 (109.6322, -41.8177) -> (122.6322, -41.8177)
  line L573 (-52.2928, -3.7177) -> (-39.2928, -3.7177)
  line L574 (176.3072, -84.9677) -> (189.3072, -84.9677)
  arc A533 (-19.7428, -9.2677) -> (-20.2428, -8.7677) centre (-20.2428, -9.2677) ccw
  arc A534 (33.4322, -27.8177) -> (32.9322, -28.3177) centre (33.4322, -28.3177) ccw
  line L575 (94.5572, 9.7823) -> (94.5572, -3.2177)
  line L576 (119.1572, -98.9677) -> (132.1572, -98.9677)
  line L577 (-71.3428, -22.7677) -> (-58.3428, -22.7677)
  arc A535 (113.1072, -98.9677) -> (113.6072, -98.4677) centre (113.1072, -98.4677) ccw
  line L578 (42.9572, -22.7677) -> (55.9572, -22.7677)
  arc A536 (62.0072, -8.7677) -> (61.5072, -9.2677) centre (62.0072, -9.2677) ccw
  arc A537 (4.3572, -22.2677) -> (4.8572, -22.7677) centre (4.8572, -22.2677) ccw
  line L579 (132.6572, -9.2677) -> (132.6572, -22.2677)
  line L580 (-38.7928, 9.7823) -> (-38.7928, -3.2177)
  arc A538 (84.0509, -100.4677) -> (84.5509, -100.9677) centre (84.5509, -100.4677) ccw
  line L581 (166.2822, -9.2677) -> (166.2822, -22.2677)
  line L582 (76.2947, -46.8677) -> (89.2947, -46.8677)
  line L583 (194.8572, -66.4177) -> (194.8572, -79.4177)
  arc A539 (85.0322, -28.3177) -> (84.5322, -27.8177) centre (84.5322, -28.3177) ccw
  line L584 (51.9822, -28.3177) -> (51.9822, -41.3177)
  arc A540 (71.0322, -41.3177) -> (71.5322, -41.8177) centre (71.5322, -41.3177) ccw
  arc A541 (89.2947, -60.8677) -> (89.7947, -60.3677) centre (89.2947, -60.3677) ccw
  arc A542 (189.8072, -66.4177) -> (189.3072, -65.9177) centre (189.3072, -66.4177) ccw
  line L585 (23.9072, -22.7677) -> (36.9072, -22.7677)
  arc A543 (-19.7428, 9.7823) -> (-20.2428, 10.2823) centre (-20.2428, 9.7823) ccw
  line L586 (132.6572, -85.4677) -> (132.6572, -98.4677)
  line L587 (189.8072, -85.4677) -> (189.8072, -98.4677)
  line L588 (100.1072, -84.9677) -> (113.1072, -84.9677)
  arc A544 (79.7697, -79.9177) -> (80.2697, -79.4177) centre (79.7697, -79.4177) ccw
  line L589 (-52.2928, 10.2823) -> (-39.2928, 10.2823)
  arc A545 (61.5072, -22.2677) -> (62.0072, -22.7677) centre (62.0072, -22.2677) ccw
  line L590 (162.4629, -48.3677) -> (162.4629, -62.3677)
  line L591 (-14.1928, -3.7177) -> (-1.1928, -3.7177)
  line L592 (155.9629, -47.8677) -> (161.9629, -47.8677)
  line L593 (100.1072, -98.9677) -> (113.1072, -98.9677)
  line L594 (-4.6678, -41.8177) -> (8.3322, -41.8177)
  line L595 (138.2072, -98.9677) -> (151.2072, -98.9677)
  arc A546 (4.3572, -3.2177) -> (4.8572, -3.7177) centre (4.8572, -3.2177) ccw
  arc A547 (75.5072, 9.7823) -> (75.0072, 10.2823) centre (75.0072, 9.7823) ccw
  arc A548 (113.6072, -85.4677) -> (113.1072, -84.9677) centre (113.1072, -85.4677) ccw
  arc A549 (27.8822, -28.3177) -> (27.3822, -27.8177) centre (27.3822, -28.3177) ccw
  line L596 (76.2947, -60.8677) -> (89.2947, -60.8677)
  arc A550 (70.2447, -60.8677) -> (70.7447, -60.3677) centre (70.2447, -60.3677) ccw
  arc A551 (55.9572, -22.7677) -> (56.4572, -22.2677) centre (55.9572, -22.2677) ccw
  line L597 (-57.8428, 9.7823) -> (-57.8428, -3.2177)
  arc A552 (80.2697, -66.4177) -> (79.7697, -65.9177) centre (79.7697, -66.4177) ccw
  arc A553 (-14.6928, -3.2177) -> (-14.1928, -3.7177) centre (-14.1928, -3.2177) ccw
  line L598 (208.8572, -66.4177) -> (208.8572, -79.4177)
  line L599 (-33.7428, 9.7823) -> (-33.7428, -3.2177)
  arc A554 (90.0822, -41.3177) -> (90.5822, -41.8177) centre (90.5822, -41.3177) ccw
  arc A555 (132.1572, -22.7677) -> (132.6572, -22.2677) centre (132.1572, -22.2677) ccw
  arc A556 (95.3447, -46.8677) -> (94.8447, -47.3677) centre (95.3447, -47.3677) ccw
  line L600 (62.0072, -3.7177) -> (75.0072, -3.7177)
  line L601 (66.7697, -65.9177) -> (79.7697, -65.9177)
  line L602 (118.6572, -85.4677) -> (118.6572, -98.4677)
  line L603 (157.8442, -10.2677) -> (157.8442, -24.2677)
  line L604 (-38.7928, -9.2677) -> (-38.7928, -22.2677)
  arc A557 (-1.1928, -3.7177) -> (-0.6928, -3.2177) centre (-1.1928, -3.2177) ccw
  arc A558 (118.6572, -98.4677) -> (119.1572, -98.9677) centre (119.1572, -98.4677) ccw
  line L605 (149.6134, -66.4177) -> (149.6134, -79.4177)
  line L606 (-76.8928, -9.2677) -> (-76.8928, -22.2677)
  arc A559 (161.2322, -28.3177) -> (160.7322, -27.8177) centre (160.7322, -28.3177) ccw
  arc A560 (103.5822, -41.8177) -> (104.0822, -41.3177) centre (103.5822, -41.3177) ccw
  line L607 (61.5072, 9.7823) -> (61.5072, -3.2177)
  arc A561 (80.5572, -3.2177) -> (81.0572, -3.7177) centre (81.0572, -3.2177) ccw
  line L608 (-33.7428, -9.2677) -> (-33.7428, -22.2677)
  arc A562 (195.3572, -65.9177) -> (194.8572, -66.4177) centre (195.3572, -66.4177) ccw
  line L609 (138.2072, -22.7677) -> (151.2072, -22.7677)
  arc A563 (-33.2428, -8.7677) -> (-33.7428, -9.2677) centre (-33.2428, -9.2677) ccw
  line L610 (113.6072, -85.4677) -> (113.6072, -98.4677)
  line L611 (-52.7928, -9.2677) -> (-52.7928, -22.2677)
  arc A564 (70.7447, -47.3677) -> (70.2447, -46.8677) centre (70.2447, -47.3677) ccw
  arc A565 (-38.7928, -9.2677) -> (-39.2928, -8.7677) centre (-39.2928, -9.2677) ccw
  line L612 (80.2697, -66.4177) -> (80.2697, -79.4177)
  line L613 (151.7072, -9.2677) -> (151.7072, -22.2677)
  arc A566 (-10.7178, -41.8177) -> (-10.2178, -41.3177) centre (-10.7178, -41.3177) ccw
  line L614 (-57.8428, -9.2677) -> (-57.8428, -22.2677)
  line L615 (71.0322, -28.3177) -> (71.0322, -41.3177)
  line L616 (195.3572, -65.9177) -> (208.3572, -65.9177)
  line L617 (65.9822, -28.3177) -> (65.9822, -41.3177)
  arc A567 (94.8447, -60.3677) -> (95.3447, -60.8677) centre (95.3447, -60.3677) ccw
  line L618 (62.0072, -8.7677) -> (75.0072, -8.7677)
  line L619 (-19.7428, 9.7823) -> (-19.7428, -3.2177)
  line L620 (-14.1928, -8.7677) -> (-1.1928, -8.7677)
  arc A568 (132.6572, -85.4677) -> (132.1572, -84.9677) centre (132.1572, -85.4677) ccw
  line L621 (-90.8928, -9.2677) -> (-90.8928, -22.2677)
  line L622 (138.2072, -84.9677) -> (151.2072, -84.9677)
  line L623 (62.0072, -22.7677) -> (75.0072, -22.7677)
  arc A569 (4.8572, 10.2823) -> (4.3572, 9.7823) centre (4.8572, 9.7823) ccw
  line L624 (-4.6678, -27.8177) -> (8.3322, -27.8177)
  arc A570 (147.2322, -41.3177) -> (147.7322, -41.8177) centre (147.7322, -41.3177) ccw
  line L625 (150.1134, -79.9177) -> (163.1134, -79.9177)
  arc A571 (128.1822, -41.3177) -> (128.6822, -41.8177) centre (128.6822, -41.3177) ccw
  arc A572 (166.2822, -22.2677) -> (166.7822, -22.7677) centre (166.7822, -22.2677) ccw
  arc A573 (137.4197, -66.4177) -> (136.9197, -65.9177) centre (136.9197, -66.4177) ccw
  arc A574 (-57.0553, -46.8677) -> (-57.5553, -47.3677) centre (-57.0553, -47.3677) ccw
  arc A575 (91.0509, -86.4677) -> (90.5509, -85.9677) centre (90.5509, -86.4677) ccw
  arc A576 (76.2947, -46.8677) -> (75.7947, -47.3677) centre (76.2947, -47.3677) ccw
  arc A577 (108.8447, -47.3677) -> (108.3447, -46.8677) centre (108.3447, -47.3677) ccw
  line L626 (85.0322, -28.3177) -> (85.0322, -41.3177)
  line L627 (84.0509, -86.4677) -> (84.0509, -100.4677)
  arc A578 (137.7072, -22.2677) -> (138.2072, -22.7677) centre (138.2072, -22.2677) ccw
  arc A579 (-5.4553, -47.3677) -> (-5.9553, -46.8677) centre (-5.9553, -47.3677) ccw
  arc A580 (-57.8428, 9.7823) -> (-58.3428, 10.2823) centre (-58.3428, 9.7823) ccw
  line L628 (66.2697, -66.4177) -> (66.2697, -79.4177)
  arc A581 (-52.7928, -3.2177) -> (-52.2928, -3.7177) centre (-52.2928, -3.2177) ccw
  arc A582 (138.2072, -84.9677) -> (137.7072, -85.4677) centre (138.2072, -85.4677) ccw
  line L629 (84.5509, -85.9677) -> (90.5509, -85.9677)
  arc A583 (8.8322, -28.3177) -> (8.3322, -27.8177) centre (8.3322, -28.3177) ccw
  line L630 (164.8442, -10.2677) -> (164.8442, -24.2677)
  line L631 (-38.0053, -46.8677) -> (-25.0053, -46.8677)
  arc A584 (127.8947, -47.3677) -> (127.3947, -46.8677) centre (127.3947, -47.3677) ccw
  arc A585 (194.8572, -60.3677) -> (195.3572, -60.8677) centre (195.3572, -60.3677) ccw
  line L632 (104.8697, -79.9177) -> (117.8697, -79.9177)
  line L633 (119.1572, -84.9677) -> (132.1572, -84.9677)
  arc A586 (-38.7928, 9.7823) -> (-39.2928, 10.2823) centre (-39.2928, 9.7823) ccw
  line L634 (71.5322, -41.8177) -> (84.5322, -41.8177)
  line L635 (-71.8428, -9.2677) -> (-71.8428, -22.2677)
  arc A587 (100.1072, -84.9677) -> (99.6072, -85.4677) centre (100.1072, -85.4677) ccw
  line L636 (-52.2928, -22.7677) -> (-39.2928, -22.7677)
  arc A588 (208.8572, -66.4177) -> (208.3572, -65.9177) centre (208.3572, -66.4177) ccw
  arc A589 (147.7322, -27.8177) -> (147.2322, -28.3177) centre (147.7322, -28.3177) ccw
  arc A590 (61.2197, -66.4177) -> (60.7197, -65.9177) centre (60.7197, -66.4177) ccw
  arc A591 (65.4822, -41.8177) -> (65.9822, -41.3177) centre (65.4822, -41.3177) ccw
  arc A592 (99.6072, -98.4677) -> (100.1072, -98.9677) centre (100.1072, -98.4677) ccw
  arc A593 (119.1572, -84.9677) -> (118.6572, -85.4677) centre (119.1572, -85.4677) ccw
  line L637 (142.1822, -28.3177) -> (142.1822, -41.3177)
  arc A594 (-5.1678, -41.3177) -> (-4.6678, -41.8177) centre (-4.6678, -41.3177) ccw
  arc A595 (150.1134, -65.9177) -> (149.6134, -66.4177) centre (150.1134, -66.4177) ccw
  arc A596 (151.2072, -22.7677) -> (151.7072, -22.2677) centre (151.2072, -22.2677) ccw
  arc A597 (-71.8428, -3.2177) -> (-71.3428, -3.7177) centre (-71.3428, -3.2177) ccw
  arc A598 (157.8442, -24.2677) -> (158.3442, -24.7677) centre (158.3442, -24.2677) ccw
  arc A599 (146.9447, -47.3677) -> (146.4447, -46.8677) centre (146.4447, -47.3677) ccw
  arc A600 (-1.1928, -22.7677) -> (-0.6928, -22.2677) centre (-1.1928, -22.2677) ccw
  line L638 (-72.1303, -28.3177) -> (-72.1303, -41.3177)
  line L639 (128.1822, -28.3177) -> (128.1822, -41.3177)
  arc A601 (-10.2178, -28.3177) -> (-10.7178, -27.8177) centre (-10.7178, -28.3177) ccw
  line L640 (109.1322, -28.3177) -> (109.1322, -41.3177)
  line L641 (-83.2491, -46.8677) -> (-70.2491, -46.8677)
  arc A602 (109.6322, -27.8177) -> (109.1322, -28.3177) centre (109.6322, -28.3177) ccw
  arc A603 (160.7322, -41.8177) -> (161.2322, -41.3177) centre (160.7322, -41.3177) ccw
  line L642 (-86.1303, -28.3177) -> (-86.1303, -41.3177)
  arc A604 (71.5322, -27.8177) -> (71.0322, -28.3177) centre (71.5322, -28.3177) ccw
  arc A605 (90.5509, -100.9677) -> (91.0509, -100.4677) centre (90.5509, -100.4677) ccw
  arc A606 (-20.2428, -22.7677) -> (-19.7428, -22.2677) centre (-20.2428, -22.2677) ccw
  arc A607 (84.5322, -41.8177) -> (85.0322, -41.3177) centre (84.5322, -41.3177) ccw
  line L643 (-5.1678, -28.3177) -> (-5.1678, -41.3177)
  line L644 (-42.7678, -41.8177) -> (-29.7678, -41.8177)
  arc A608 (-76.8928, 9.7823) -> (-77.3928, 10.2823) centre (-77.3928, 9.7823) ccw
  line L645 (155.4629, -48.3677) -> (155.4629, -62.3677)
  arc A609 (-24.5053, -47.3677) -> (-25.0053, -46.8677) centre (-25.0053, -47.3677) ccw
  line L646 (-48.3178, -28.3177) -> (-48.3178, -41.3177)
  arc A610 (133.4447, -46.8677) -> (132.9447, -47.3677) centre (133.4447, -47.3677) ccw
  line L647 (-24.2178, -28.3177) -> (-24.2178, -41.3177)
  arc A611 (18.6447, -60.3677) -> (19.1447, -60.8677) centre (19.1447, -60.3677) ccw
  arc A612 (177.4009, -60.8677) -> (177.9009, -60.3677) centre (177.4009, -60.3677) ccw
  line L648 (75.5072, 9.7823) -> (75.5072, -3.2177)
  arc A613 (-33.7428, -3.2177) -> (-33.2428, -3.7177) centre (-33.2428, -3.2177) ccw
  line L649 (-0.6928, -9.2677) -> (-0.6928, -22.2677)
  line L650 (91.0509, -86.4677) -> (91.0509, -100.4677)
  arc A614 (32.9322, -41.3177) -> (33.4322, -41.8177) centre (33.4322, -41.3177) ccw
  line L651 (195.3572, -84.9677) -> (208.3572, -84.9677)
  line L652 (195.3572, -79.9177) -> (208.3572, -79.9177)
  arc A615 (151.7072, -9.2677) -> (151.2072, -8.7677) centre (151.2072, -9.2677) ccw
  line L653 (-78.4866, -79.9177) -> (-65.4866, -79.9177)
  arc A616 (138.2072, 10.2823) -> (137.7072, 9.7823) centre (138.2072, 9.7823) ccw
  arc A617 (175.8072, -98.4677) -> (176.3072, -98.9677) centre (176.3072, -98.4677) ccw
  arc A618 (94.0572, -3.7177) -> (94.5572, -3.2177) centre (94.0572, -3.2177) ccw
  arc A619 (104.8697, -65.9177) -> (104.3697, -66.4177) centre (104.8697, -66.4177) ccw
  arc A620 (-0.6928, -9.2677) -> (-1.1928, -8.7677) centre (-1.1928, -9.2677) ccw
  arc A621 (163.6134, -66.4177) -> (163.1134, -65.9177) centre (163.1134, -66.4177) ccw
  line L654 (-40.3866, -84.9677) -> (-27.3866, -84.9677)
  line L655 (9.1197, -66.4177) -> (9.1197, -79.4177)
  line L656 (118.6572, 9.7823) -> (118.6572, -3.2177)
  line L657 (179.3389, -48.3677) -> (179.3389, -62.3677)
  line L658 (32.9322, -28.3177) -> (32.9322, -41.3177)
  line L659 (208.8572, -85.4677) -> (208.8572, -98.4677)
  line L660 (-14.9803, -66.4177) -> (-14.9803, -79.4177)
  arc A622 (137.7072, -98.4677) -> (138.2072, -98.9677) centre (138.2072, -98.4677) ccw
  line L661 (189.8072, -66.4177) -> (189.8072, -79.4177)
  line L662 (123.4197, -66.4177) -> (123.4197, -79.4177)
  arc A623 (104.3697, -79.4177) -> (104.8697, -79.9177) centre (104.8697, -79.4177) ccw
  arc A624 (36.9072, -22.7677) -> (37.4072, -22.2677) centre (36.9072, -22.2677) ccw
  line L663 (-52.7928, 9.7823) -> (-52.7928, -3.2177)
  line L664 (42.4572, -9.2677) -> (42.4572, -22.2677)
  arc A625 (90.5822, -27.8177) -> (90.0822, -28.3177) centre (90.5822, -28.3177) ccw
  arc A626 (208.3572, -98.9677) -> (208.8572, -98.4677) centre (208.3572, -98.4677) ccw
  arc A627 (151.7072, -85.4677) -> (151.2072, -84.9677) centre (151.2072, -85.4677) ccw
  arc A628 (166.7822, -8.7677) -> (166.2822, -9.2677) centre (166.7822, -9.2677) ccw
  arc A629 (-9.4491, -100.9677) -> (-8.9491, -100.4677) centre (-9.4491, -100.4677) ccw
  arc A630 (-26.8866, -85.4677) -> (-27.3866, -84.9677) centre (-27.3866, -85.4677) ccw
  line L665 (19.1447, -46.8677) -> (32.1447, -46.8677)
  line L666 (104.8697, -65.9177) -> (117.8697, -65.9177)
  arc A631 (-78.9866, -79.4177) -> (-78.4866, -79.9177) centre (-78.4866, -79.4177) ccw
  line L667 (33.4322, -41.8177) -> (46.4322, -41.8177)
  arc A632 (208.3572, -60.8677) -> (208.8572, -60.3677) centre (208.3572, -60.3677) ccw
  line L668 (-78.4866, -65.9177) -> (-65.4866, -65.9177)
  arc A633 (-50.6991, -85.4677) -> (-51.1991, -84.9677) centre (-51.1991, -85.4677) ccw
  arc A634 (27.3822, -41.8177) -> (27.8822, -41.3177) centre (27.3822, -41.3177) ccw
  arc A635 (113.6072, -9.2677) -> (113.1072, -8.7677) centre (113.1072, -9.2677) ccw
  arc A636 (-48.0303, -79.4177) -> (-47.5303, -79.9177) centre (-47.5303, -79.4177) ccw
  line L669 (46.9322, -28.3177) -> (46.9322, -41.3177)
  arc A637 (-20.2428, -3.7177) -> (-19.7428, -3.2177) centre (-20.2428, -3.2177) ccw
  line L670 (4.0697, -66.4177) -> (4.0697, -79.4177)
  arc A638 (75.7947, -60.3677) -> (76.2947, -60.8677) centre (76.2947, -60.3677) ccw
  arc A639 (4.0697, -66.4177) -> (3.5697, -65.9177) centre (3.5697, -66.4177) ccw
  arc A640 (194.8572, -98.4677) -> (195.3572, -98.9677) centre (195.3572, -98.4677) ccw
  line L671 (80.5572, 9.7823) -> (80.5572, -3.2177)
  line L672 (4.3572, 9.7823) -> (4.3572, -3.2177)
  line L673 (27.8822, -28.3177) -> (27.8822, -41.3177)
  line L674 (-63.0486, -66.9177) -> (-57.0486, -66.9177)
  arc A641 (61.5072, -3.2177) -> (62.0072, -3.7177) centre (62.0072, -3.2177) ccw
  arc A642 (-51.1991, -98.9677) -> (-50.6991, -98.4677) centre (-51.1991, -98.4677) ccw
  line L675 (-8.9491, -86.4677) -> (-8.9491, -100.4677)
  line L676 (175.8072, -66.4177) -> (175.8072, -79.4177)
  arc A643 (84.5509, -85.9677) -> (84.0509, -86.4677) centre (84.5509, -86.4677) ccw
  arc A644 (94.5572, -9.2677) -> (94.0572, -8.7677) centre (94.0572, -9.2677) ccw
  line L677 (166.7822, -22.7677) -> (179.7822, -22.7677)
  line L678 (176.3072, -98.9677) -> (189.3072, -98.9677)
  line L679 (66.7697, -79.9177) -> (79.7697, -79.9177)
  line L680 (195.3572, -60.8677) -> (208.3572, -60.8677)
  arc A645 (-14.1928, 10.2823) -> (-14.6928, 9.7823) centre (-14.1928, 9.7823) ccw
  arc A646 (100.1072, 10.2823) -> (99.6072, 9.7823) centre (100.1072, 9.7823) ccw
  arc A647 (81.0572, 10.2823) -> (80.5572, 9.7823) centre (81.0572, 9.7823) ccw
  line L681 (-0.6928, 9.7823) -> (-0.6928, -3.2177)
  line L682 (137.7072, -9.2677) -> (137.7072, -22.2677)
  line L683 (157.2572, -98.9677) -> (170.2572, -98.9677)
  line L684 (179.8389, -62.8677) -> (185.8389, -62.8677)
  arc A648 (62.0072, 10.2823) -> (61.5072, 9.7823) centre (62.0072, 9.7823) ccw